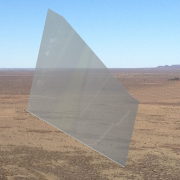
# Autodesk Inventor part: 2r4scr
Saved by Autodesk Inventor 2013 SP2 (Build 170200200, 200)
## iProperties
Company: HERA Project
Created: 2013-12-16
Part Number: 2r4scr
Material: Glass
Document SubType Name: Modeling
Designer: David DeBoer
Mass: 98383.3 g
Surface Area: 143280 cm^2
Volume: 45130 cm^3
Density: 2.18 g/cm^3
Description: screen - right
Author: David DeBoer
Autodesk Inventor part; units mm, degrees
ref_plane "YZ Plane" through (0, 0, 0) normal (1, 0, 0) x (0, 1, 0)
sketch "Sketch1" plane through (0, 0, 0) normal (0, 1, 0) x (-1, 0, 0)
  line L0 (0, 0) -> (-3454.4, 0)
  line L1 (-3454.4, 0) -> (-3454.4, -25.4)
  line L2 (-3454.4, -25.4) -> (0, -25.4)
  line L3 (0, -25.4) -> (0, 0)
  dimension "d0" = 3454.4
  dimension "d1" = 25.4
  constraints: 8 end point, 2 parallel, 1 horizontal, 1 perpendicular
  measures "d0" distance of L0.start L0.end
  measures "d1" distance of L2.end L0.start
extrude "base" add sketch "Sketch1" along normal blind 6.35
ref_plane "right" through (3454.4, 6.35, -25.4) normal (0, 0.9925462, -0.1218693) x (-1, 0, 0)
sketch "Sketch7" plane through (3454.4, 6.35, -25.4) normal (0, 0.9925462, -0.1218693) x (-1, 0, 0)
  line L0 (0, 0) -> (12.7, 0)
  line L1 (12.7, 0) -> (12.7, 6.35)
  line L2 (12.7, 6.35) -> (0, 6.35)
  line L3 (0, 6.35) -> (0, 0)
  point P0 (3454.4, 24.4368)
  constraints: 8 end point, 2 parallel, 1 horizontal, 1 perpendicular
extrude "upRight" add sketch "Sketch7" along normal blind 2032
sketch "Sketch8" plane through (3454.4, 7.1239, -19.0973) normal (0, 0.1218693, 0.9925462) x (1, 0, 0)
  line L0 (0, 0) -> (0, 2032) projected
  line L1 (-12.7, 0) -> (-12.7, 2032) projected
  line L2 (0, 2032) -> (254, 2032)
  line L3 (254, 2032) -> (0, 0)
  point P0 (-3454.4, -9.3981)
  dimension "d36" = 254
  constraints: 4 end point, 1 perpendicular
  measures "d36" distance of L0.end L2.end
extrude "outRight" add sketch "Sketch8" against normal blind 6.35
ref_plane "left" through (3454.4, 6.35, -25.4) normal (0, 0.8660254, -0.5) x (-1, 0, 0)
sketch "Sketch9" plane through (3454.4, 6.35, -25.4) normal (0, 0.8660254, -0.5) x (-1, 0, 0)
  line L0 (3454.4, 0) -> (3441.7, 0)
  line L1 (3441.7, 0) -> (3441.7, 6.35)
  line L2 (3441.7, 6.35) -> (3454.4, 6.35)
  line L3 (3454.4, 6.35) -> (3454.4, 0)
  point P0 (3454.4, 18.822)
  dimension "d40" = 12.7
  dimension "d41" = 6.35
  constraints: 8 end point, 2 parallel, 1 horizontal, 1 perpendicular
  measures "d40" distance of L1.end L2.end
  measures "d41" distance of L0.end L1.end
extrude "upLeft" add sketch "Sketch9" along normal blind 2540
sketch "Sketch10" plane through (12.7, 9.525, -19.9007) normal (0, 0.5, 0.8660254) x (1, 0, 0)
  line L0 (-12.7, 0) -> (-12.7, 2540) projected
  line L1 (-12.7, 2540) -> (-520.7, 2540)
  line L2 (-520.7, 2540) -> (-12.7, 0)
  point P0 (-12.7, -18.1993)
  dimension "d44" = 508
  constraints: 4 end point, 1 perpendicular
  measures "d44" distance of L0.end L1.end
extrude "outLeft" add sketch "Sketch10" against normal blind 6.35
loft "Loft3" add section 1 edges at (12.7, 7.9375, -22.6504) (12.7, 1106.2023, -660.4) (12.7, 2207.642, -1292.6504) (12.7, 1109.3773, -654.9007) section 2 edges at (3441.7, 6.7369, -22.2487) (3441.7, 1015.5508, -142.9166) (3441.7, 2023.5907, -269.8872) (3441.7, 1014.7769, -149.2193)
body "Solid1"
